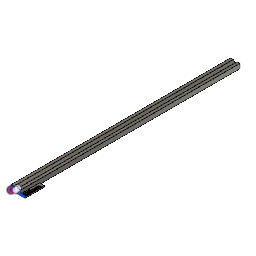
jig_cable_230mm (Autodesk Fusion 360 design; units mm, degrees)
Autodesk Fusion 360 part; units mm, degrees
sketch "スケッチ1" plane through (0, 0, 0) normal (0, 0, 1) x (1, 0, 0)
  line L0 (0, 5) -> (10, 5)
  line L1 (10, 5) -> (10, 0)
  line L2 (10, 0) -> (0, 0)
  line L3 (0, 0) -> (0, 5)
  line L4 (5, 5) -> (5, 0)
  line L5 (5, 2.5) -> (3, 5)
  line L6 (5, 2.5) -> (7, 5)
  line L7 (10, 0) -> (15, 0)
  line L8 (15, 0) -> (15, 1.5)
  line L9 (15, 1.5) -> (10, 1.5)
  line L10 (10, 1.5) -> (10, 0)
  line L11 (0, 0) -> (10, 0)
  line L12 (10, 0) -> (10, 4.5)
  line L13 (10, 4.5) -> (0, 4.5)
  line L14 (0, 4.5) -> (0, 0)
  dimension "d3" = 1.5
  dimension "d4" = 5
  dimension "d7" = 4.5
  constraint horizontal L0
  constraint vertical L1
  constraint horizontal L2
  constraint vertical L3
  constraint midpoint L0 L4.start
  constraint midpoint L2 L4.end
  constraint midpoint L4 L5.start
  constraint coincident L0 L5.end
  constraint symmetric L4 L5.start L6.start
  constraint symmetric L4 L5.end L6.end
  constraint horizontal L7
  constraint vertical L8
  constraint horizontal L9
  constraint vertical L10
  constraint horizontal L11
  constraint vertical L12
  constraint horizontal L13
  constraint vertical L14
  constraint coincident L2.end L3.start
  measures "d3" distance of L1.end L9.end
  measures "d4" distance of L1.end L7.end
  measures "d7" distance of L2.end L13.end
extrude "押し出し1" add sketch "スケッチ1" against normal blind 230 contours L0 L3 L5 L13 | L2 L3 L4 L5 L11 L13 L14 | L0 L1 L6 L13 | L1 L2 L4 L6 L10 L11 L12 L13 makes body 1
extrude "押し出し2" add sketch "スケッチ1" against normal blind 50 contours L1 L7 L8 L9 L10 L12 bodies 1
sketch "スケッチ2" plane through (0, 0, 0) normal (0, 1, 0) x (1, 0, 0)
  line L0 (14.5, 0.5) -> (14.5, 17.2847) construction
  line L1 (14.5, 17.2847) -> (9.5, 17.2847) construction
  line L2 (9.5, 17.2847) -> (9.5, 0.5) construction
  line L3 (9.5, 0.5) -> (14.5, 0.5) construction
  text T0 "230mm" font "Arial" height 5 bold align ink ink in box 0 x 0 at (14.48, 0.51) x (0, 1) y (-1, 0) spacing 1 height is em
  constraint perpendicular L0 L1
  constraint parallel L0 L2
  constraint parallel L1 L3
extrude "押し出し3" cut sketch "スケッチ2" along normal blind 3 text T0 bodies 1 makes body 2 at (12.3589, 1.5, -7.1716)
extrude "押し出し4" add sketch "スケッチ2" along normal blind 1 text T0 bodies 1 2
extrude "押し出し5" cut 1 faces at (11.6667, 1, -50) along direction (0, 0, 1) blind 30 on bodies 1 bodies 1
